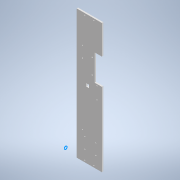
# Autodesk Inventor part: top of drivetrain 2
Saved by Autodesk Inventor 2020 (Build 240168000, 168)
## iProperties
Created: 2020-03-07
Part Number: top of drivetrain 2
Material: Generic
Document SubType Name: Modeling
Designer: jackm
Density: 1 g/cm^3
Appearance: Default
Author: jackm
Autodesk Inventor part; units mm, degrees
ref_plane "YZ Plane" through (0, 0, 0) normal (1, 0, 0) x (0, 1, 0)
ref_plane "XZ Plane" through (0, 0, 0) normal (0, 1, 0) x (-1, 0, 0)
ref_plane "XY Plane" through (0, 0, 0) normal (0, 0, 1) x (1, 0, 0)
ref_plane "Work Plane1" through (0, 0, 0) normal (0, 0, 1) x (0, -1, 0)
sketch "Sketch1" plane through (0, 0, 0) normal (0, 0, 1) x (0, -1, 0)
  line L0 (-450.85, 82.6732) -> (0, 82.6732) construction
  line L1 (0, -5) -> (-450.85, -5) construction
  line L2 (-450.85, -5) -> (-450.85, 82.6732)
  line L3 (0, 82.6732) -> (0, -5)
  line L4 (0, -5) -> (-450.85, -5)
  circle A0 centre (-444.5, 22.86) radius 1.7 construction
  circle A1 centre (-444.5, 54.8132) radius 1.7 construction
  circle A2 centre (-252.8255, 65.525) radius 1.9304 construction
  circle A3 centre (-210.0251, 65.525) radius 1.9304 construction
  circle A4 centre (-6.35, 54.8132) radius 1.7 construction
  circle A5 centre (-6.35, 22.86) radius 1.7 construction
  circle A6 centre (-94.9, 14.5) radius 1.7 construction
  circle A7 centre (-349.219, 14.5) radius 1.7 construction
  circle A8 centre (-444.5, 22.86) radius 1.7
  circle A9 centre (-444.5, 54.8132) radius 1.7
  circle A10 centre (-349.219, 14.5) radius 1.7
  circle A11 centre (-252.8255, 65.525) radius 1.7
  circle A12 centre (-210.0251, 65.525) radius 1.7
  circle A13 centre (-94.9, 14.5) radius 1.7
  circle A14 centre (-6.35, 54.8132) radius 1.7
  circle A15 centre (-6.35, 22.86) radius 1.7
  circle A16 centre (-78.0653, 61.3428) radius 1.7
  line L5 (-78.0653, 61.3428) -> (-78.0653, 23.2428) construction
  line L6 (-78.0653, 23.2428) -> (-39.9653, 23.2428) construction
  line L7 (-39.9653, 23.2428) -> (-39.9653, 61.3428) construction
  circle A17 centre (-78.0653, 23.2428) radius 1.7
  circle A18 centre (-39.9653, 23.2428) radius 1.7
  circle A19 centre (-39.9653, 61.3428) radius 1.7
  line L8 (-450.85, 15.32) -> (-311.15, 15.32) construction
  circle A20 centre (-311.15, 15.32) radius 1.7
  line L9 (-241.6818, 27.8034) -> (-231.5218, 27.8034)
  line L10 (-231.5218, 27.8034) -> (-231.5218, 37.9634)
  line L11 (-231.5218, 37.9634) -> (-241.6818, 37.9634)
  line L12 (-241.6818, 37.9634) -> (-241.6818, 27.8034)
  line L13 (-349.219, 82.6732) -> (-349.219, 57.2732)
  line L14 (-349.219, 57.2732) -> (-257.779, 57.2732)
  line L15 (-257.779, 57.2732) -> (-257.779, 82.6732)
  circle A21 centre (-276.829, 48.7923) radius 1.7
  circle A22 centre (-330.169, 48.7923) radius 1.7
  line L16 (-450.85, 82.6732) -> (-349.219, 82.6732)
  line L17 (-257.779, 82.6732) -> (0, 82.6732)
  point P0 (0, 0)
  dimension "d0" = 3.4
  dimension "d1" = 3.4
  dimension "d2" = 3.4
  dimension "d3" = 3.4
  dimension "d4" = 3.4
  dimension "d5" = 3.4
  dimension "d6" = 3.4
  dimension "d7" = 3.4
  dimension "d8" = 3.4
  dimension "d9" = 38.1
  dimension "d10" = 38.1
  dimension "d11" = 38.1
  dimension "d12" = 3.4
  dimension "d13" = 3.4
  dimension "d14" = 3.4
  dimension "d21" = 139.7
  dimension "d22" = 20.32
  dimension "d23" = 3.4
  dimension "d24" = 10.16
  dimension "d25" = 10.16
  dimension "d26" = 25.4
  dimension "d27" = 91.44
  dimension "d28" = 3.4
  dimension "d29" = 3.4
  dimension "d30" = 19.05
  dimension "d31" = 19.05
  constraints: 32 end point, 15 centre point, 12 coincident, 11 perpendicular, 3 equal length, 2 vertical, 1 horizontal, 1 point on line
  measures "d0" diameter of A8
  measures "d1" diameter of A9
  measures "d2" diameter of A10
  measures "d3" diameter of A11
  measures "d4" diameter of A12
  measures "d5" diameter of A13
  measures "d6" diameter of A14
  measures "d7" diameter of A15
  measures "d8" diameter of A16
  measures "d9" distance of L5.start L5.end
  measures "d10" distance of L5.end L6.end
  measures "d11" distance of L6.end L7.end
  measures "d12" diameter of A17
  measures "d13" diameter of A18
  measures "d14" diameter of A19
  measures "d21" distance of L8.start L8.end
  measures "d22" distance between parallel lines of L1 L8
  measures "d23" diameter of A20
  measures "d24" distance of L11.end L10.end
  measures "d25" distance of L10.end L9.end
  measures "d26" distance of L13.start L13.end
  measures "d27" distance of L13.end L14.end
  measures "d28" diameter of A21
  measures "d29" diameter of A22
  measures "d30" distance from line of L15 A21.centre
  measures "d31" distance from line of L13 A22.centre
extrude "Extrusion1" add sketch "Sketch1" along normal blind 5
equation "\"d31\" = d30"
body "Solid1"
